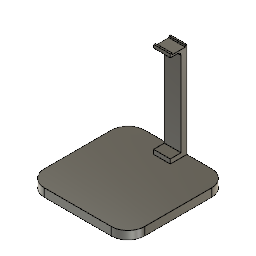
headphone stand v3 (Autodesk Fusion 360 design; units mm, degrees)
Autodesk Fusion 360 part; units mm, degrees
sketch "base" plane through (0, 0, 0) normal (0, 0, 1) x (1, 0, 0)
  line L0 (-20, 30) -> (20, 30)
  line L1 (30, 20) -> (30, -20)
  line L2 (20, -30) -> (-20, -30)
  line L3 (-30, -20) -> (-30, 20)
  line L4 (-30, 30) -> (30, -30) construction
  line L5 (30, 30) -> (-30, -30) construction
  arc A0 (-20, 30) -> (-30, 20) centre (-20, 20) ccw
  arc A1 (30, 20) -> (20, 30) centre (20, 20) ccw
  arc A2 (20, -30) -> (30, -20) centre (20, -20) ccw
  arc A3 (-30, -20) -> (-20, -30) centre (-20, -20) ccw
  dimension "d1" = 10
  dimension "d2" = 40
  dimension "d3" = 40
  constraint horizontal L0
  constraint perpendicular L0 L1
  constraint parallel L0 L2
  constraint parallel L1 L3
  constraint coincident L4 origin
  constraint coincident L5 origin
  constraint coincident L4.start L0
  constraint coincident L4.start L3
  constraint tangent L0 A0
  constraint tangent L3 A0
  constraint coincident L5.start L0
  constraint coincident L5.start L1
  constraint tangent L0 A1
  constraint tangent L1 A1
  constraint equal A0 A1
  constraint coincident L4.end L1
  constraint coincident L4.end L2
  constraint tangent L1 A2
  constraint tangent L2 A2
  constraint equal A0 A2
  constraint coincident L5.end L2
  constraint coincident L5.end L3
  constraint tangent L2 A3
  constraint tangent L3 A3
  constraint equal A0 A3
  measures "d1" radius of A0
  measures "d2" distance of A2.centre A3.centre
  measures "d3" distance of A0.centre A3.centre
extrude "Extrude1" add sketch "base" along normal blind 5
sketch "post anchor" plane through (0, 0, 5) normal (0, 0, 1) x (-1, 0, 0)
  arc A0 (20, -30) -> (30, -20) centre (20, -20) ccw
  line L0 (30, -20) -> (30, 20)
  arc A1 (30, 20) -> (20, 30) centre (20, 20) ccw
  line L1 (20, 30) -> (-20, 30)
  arc A2 (-20, 30) -> (-30, 20) centre (-20, 20) ccw
  line L2 (-30, 20) -> (-30, -20)
  arc A3 (-30, -20) -> (-20, -30) centre (-20, -20) ccw
  line L3 (-20, -30) -> (20, -30)
  line L4 (4.7066, -30) -> (-5.2934, -30)
  line L5 (4.7066, -30) -> (4.7066, -20)
  line L6 (4.7066, -20) -> (-5.2934, -20)
  line L7 (-5.2934, -20) -> (-5.2934, -30)
  point P0 (0, -30)
  dimension "d6" = 10
  dimension "d7" = 10
  constraint midpoint L3 P0
  constraint coincident L3 L4.start
  constraint coincident L3 L4.end
  constraint parallel L3 L4
  constraint perpendicular L3 L5
  constraint perpendicular L5 L6
  constraint perpendicular L6 L7
  measures "d6" distance of L5 L7
  measures "d7" distance of L4.end L6.end
extrude "Extrude2" add sketch "post anchor" along normal blind 57 contours L3 L4 L5 L6 L7
sketch "stand profile" plane through (5.2934, 0, 0) normal (1, 0, 0) x (0, 1, 0)
  line L0 (20, 5) -> (30, 5)
  line L1 (30, 5) -> (30, 62)
  line L2 (30, 62) -> (20, 62)
  line L3 (20, 62) -> (20, 5)
  line L4 (20, 5) -> (30, 5)
  line L5 (30, 62) -> (20, 62)
  line L6 (20, 59.97) -> (24.4513, 59.97)
  line L7 (26.4513, 57.97) -> (26.4513, 7.6053)
  line L8 (26.4513, 7.6053) -> (20, 7.6053)
  line L9 (20, 5) -> (20, 7.6053)
  line L10 (20, 62) -> (20, 59.97)
  arc A0 (26.4513, 57.97) -> (24.4513, 59.97) centre (24.4513, 57.97) ccw
  dimension "d10" = 3.5487
  dimension "d11" = 2.6053
  dimension "d12" = 2.03
  dimension "d13" = 2
  constraint coincident L0.start L3.end
  constraint coincident L0.end L1.start
  constraint coincident L1.end L2.start
  constraint coincident L2.end L3.start
  constraint coincident L3 L6.start
  constraint perpendicular L3 L6
  constraint perpendicular L6 L7
  constraint coincident L3 L8.end
  constraint perpendicular L3 L8
  constraint tangent L6 A0
  constraint tangent L7 A0
  measures "d10" distance of L1 L7
  measures "d11" distance of L4 L8
  measures "d12" distance of L5 L6
  measures "d13" radius of A0
extrude "Extrude3" cut sketch "stand profile" against normal blind 10 contours L3 L6 L7 L8 A0
sketch "headphone rest" plane through (5.2934, 0, 0) normal (1, 0, 0) x (0, 1, 0)
  line L0 (26.4513, 7.6053) -> (20, 7.6053)
  line L1 (20, 7.6053) -> (20, 5)
  line L2 (20, 5) -> (30, 5)
  line L3 (30, 5) -> (30, 62)
  line L4 (30, 62) -> (20, 62)
  line L5 (20, 62) -> (20, 59.97)
  line L6 (20, 59.97) -> (24.4513, 59.97)
  arc A0 (26.4513, 57.97) -> (24.4513, 59.97) centre (24.4513, 57.97) ccw
  line L7 (26.4513, 57.97) -> (26.4513, 7.6053)
  line L8 (21, 62) -> (21, 61)
  line L9 (21, 61) -> (29, 61)
  line L10 (29, 61) -> (29, 62)
  line L11 (30, 62) -> (30, 60.477)
  line L12 (20, 60.477) -> (20, 62)
  line L13 (21, 62) -> (20, 62)
  line L14 (20, 60.477) -> (30, 60.477)
  dimension "d16" = 1
  dimension "d17" = 1
  dimension "d18" = 0.523
  dimension "d19" = 1
  constraint coincident L4 L8.start
  constraint perpendicular L4 L8
  constraint perpendicular L8 L9
  constraint coincident L4 L10.end
  constraint perpendicular L4 L10
  constraint coincident L3.end L4.start
  constraint coincident L3 L11.end
  constraint perpendicular L4 L11
  constraint coincident L5 L12.start
  constraint coincident L4.end L5.start
  constraint perpendicular L4 L12
  constraint perpendicular L5 L13
  constraint perpendicular L5 L14
  measures "d16" distance of L4 L9
  measures "d17" distance of L10 L11
  measures "d18" distance of L9 L14
  measures "d19" distance of L8 L12
extrude "Extrude4" cut sketch "headphone rest" against normal blind 10 contours L4 L8 L9 L10
